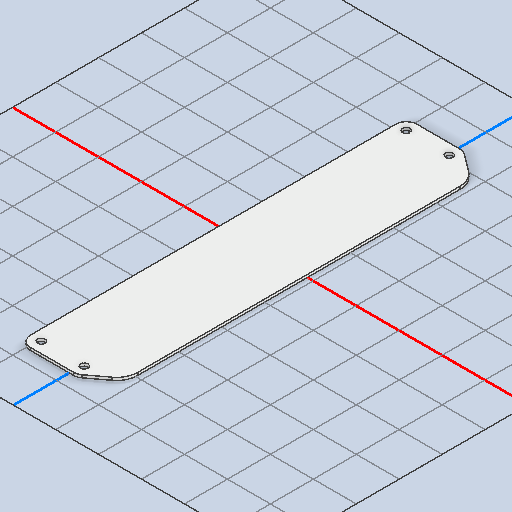
# Autodesk Inventor part: Wedge
Saved by Autodesk Inventor 2026 (Build 300175000, 175)
## iProperties
Created: 2025-04-12
Part Number: Wedge
Material: Acetal Resin, White
Document SubType Name: Modeling
Designer: avere
Density: 1.425 g/cm^3
Appearance: Smooth - White
Author: avere
Autodesk Inventor part; units mm, degrees
ref_plane "YZ Plane" through (0, 0, 0) normal (1, 0, 0) x (0, 1, 0)
ref_plane "XZ Plane" through (0, 0, 0) normal (0, 1, 0) x (-1, 0, 0)
ref_plane "XY Plane" through (0, 0, 0) normal (0, 0, 1) x (1, 0, 0)
sketch "Sketch1" plane through (0, 0, 0) normal (0, 1, 0) x (-1, 0, 0)
  circle A0 centre (-2.8921, -102.8959) radius 2.1844
  circle A1 centre (22.5079, -102.8959) radius 2.1844
  circle A2 centre (-2.8921, 113.0041) radius 2.1844
  circle A3 centre (22.5079, 113.0041) radius 2.1844
  arc A4 (28.8579, 113.0041) -> (22.5079, 119.3541) centre (22.5079, 113.0041) ccw
  arc A5 (-2.8921, 119.3541) -> (-6.7021, 118.0841) centre (-2.8921, 113.0041) ccw
  arc A6 (-6.7021, -107.9759) -> (-2.8921, -109.2459) centre (-2.8921, -102.8959) ccw
  arc A7 (22.5079, -109.2459) -> (28.8579, -102.8959) centre (22.5079, -102.8959) ccw
  line L0 (-2.8921, 119.3541) -> (22.5079, 119.3541)
  line L1 (28.8579, 113.0041) -> (28.8579, -102.8959)
  line L2 (22.5079, -109.2459) -> (-2.8921, -109.2459)
  line L3 (-16.8621, 110.4641) -> (-6.7021, 118.0841)
  line L4 (-16.8621, -100.3559) -> (-6.7021, -107.9759)
  line L5 (-21.9421, 100.3041) -> (-21.9421, -90.1959)
  arc A8 (-16.8621, 110.4641) -> (-21.9421, 100.3041) centre (-9.2421, 100.3041) ccw
  arc A9 (-21.9421, -90.1959) -> (-16.8621, -100.3559) centre (-9.2421, -90.1959) ccw
  line L6 (-2.8921, 119.3541) -> (22.5079, 119.3541)
  line L7 (22.5079, -109.2459) -> (-2.8921, -109.2459)
  line L8 (28.8579, 113.0041) -> (28.8579, -102.8959)
  point P0 (0, 0)
  dimension "d0" = 12.7
  dimension "d1" = 12.7
  dimension "d2" = 12.7
  dimension "d3" = 12.7
  constraints: 18 end point, 12 point on circle, 11 tangent, 10 centre point, 4 coincident, 2 vertical, 1 equal radius, 1 perpendicular
  measures "d0" diameter of A4
  measures "d1" diameter of A5
  measures "d2" diameter of A6
  measures "d3" radius of A8
extrude "Extrusion1" add sketch "Sketch1" along normal blind 1.5875
body "Solid1"
